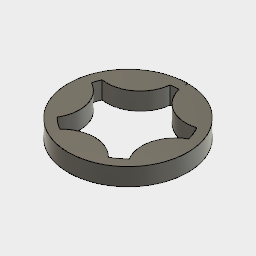
!-2 (Autodesk Fusion 360 archive; units mm, degrees)
design "模型2"
Autodesk Fusion 360 part; units mm, degrees
sketch "草图1" plane through (0, 0, 0) normal (0, 1, 0) x (1, 0, 0)
  circle A0 centre (-14.9262, -11.5502) radius 34
  arc A1 (-41.0535, -0.1653) -> (-19.1609, 16.6334) centre (-38.0591, 18.5972) ccw
  arc A2 (-35.4429, -31.3319) -> (-42.585, -4.6771) centre (-51.6314, -21.3853) ccw
  arc A3 (-1.1287, -36.4877) -> (-28.7237, -36.4877) centre (-14.9262, -49.5502) ccw
  arc A4 (12.7326, -4.6771) -> (5.5905, -31.3319) centre (21.779, -21.3853) ccw
  arc A5 (-41.0535, -0.1653) -> (-42.585, -4.6771) centre (-14.9262, -11.5502) ccw
  arc A6 (-14.4065, 16.9451) -> (-19.1609, 16.6334) centre (-14.9262, -11.5502) ccw
  arc A7 (12.7326, -4.6771) -> (9.4915, 3.1476) centre (-14.9262, -11.5502) ccw
  line L0 (-14.9262, 22.4498) -> (-14.9262, 21.3588)
  arc A8 (-14.8949, 22.4498) -> (-14.9262, 21.3588) centre (4.0738, 21.3588) ccw
  arc A9 (-14.4065, 16.9451) -> (9.4915, 3.1476) centre (4.0738, 21.3588) ccw
  arc A10 (-35.4429, -31.3319) -> (-28.7237, -36.4877) centre (-14.9262, -11.5502) ccw
  arc A11 (-1.1287, -36.4877) -> (5.5905, -31.3319) centre (-14.9262, -11.5502) ccw
  dimension "d1" = 68
  dimension "d3" = 57
  dimension "d4" = 38
  dimension "d6" = 38
  dimension "d7" = 38
  dimension "d8" = 38
  measures "d1" diameter of A0
  measures "d3" diameter of A10
  measures "d4" diameter of A3
  measures "d6" diameter of A4
  measures "d7" diameter of A8
  measures "d8" diameter of A1
extrude "拉伸1" add sketch "草图1" along normal blind 10 contours A0 L0 A8 picked at (13.385, -17.6951)
